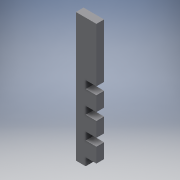
# Autodesk Inventor part: B
Saved by Autodesk Inventor 2019 (Build 230136000, 136)
## iProperties
Created: 2020-03-27
Part Number: B
Material: Generic
Document SubType Name: Modeling
Designer: Pulag
Density: 1 g/cm^3
Appearance: Default
Author: Pulag
Autodesk Inventor part; units mm, degrees
ref_plane "YZ Plane" through (0, 0, 0) normal (1, 0, 0) x (0, 1, 0)
ref_plane "XZ Plane" through (0, 0, 0) normal (0, 1, 0) x (-1, 0, 0)
ref_plane "XY Plane" through (0, 0, 0) normal (0, 0, 1) x (1, 0, 0)
sketch "Sketch1" plane through (0, 0, 0) normal (0, 0, 1) x (1, 0, 0)
  circle A0 centre (-2.5, 4.3301) radius 1.5 projected
  circle A1 centre (-2.5, -4.3301) radius 1.5 projected
  line L0 (-3.5898, 5.3609) -> (2.6004, 5.3609) construction
  line L1 (-2.5, -2.8301) -> (-6.6848, -2.8301)
  line L2 (-6.6848, -2.8301) -> (-6.6848, -5.8301)
  line L3 (-2.5, 5.8301) -> (-6.6848, 5.8301)
  line L4 (-2.5, 2.8301) -> (-6.6848, 2.8301)
  line L5 (-6.6848, 2.8301) -> (-6.6848, 5.8301)
  line L6 (-10.5, 44.1699) -> (-2.5, 44.1699)
  line L7 (-6.6848, -5.8301) -> (-10.5, -5.8301)
  line L8 (-10.5, -5.8301) -> (-10.5, 44.1699)
  line L9 (-6.6848, 0.0001) -> (-6.6849, 0)
  line L10 (-2.5, 2.8301) -> (-2.5, -2.8301)
  line L11 (-2.5, 14.4904) -> (-6.6848, 14.4904)
  line L12 (-2.5, 11.4904) -> (-6.6848, 11.4904)
  line L13 (-6.6848, 11.4904) -> (-6.6848, 14.4904)
  line L14 (-2.5, 11.4904) -> (-2.5, 5.8301)
  line L15 (-2.5, 23.1506) -> (-6.6848, 23.1506)
  line L16 (-2.5, 20.1506) -> (-6.6848, 20.1506)
  line L17 (-6.6848, 20.1506) -> (-6.6848, 23.1506)
  line L18 (-2.5, 20.1506) -> (-2.5, 14.4904)
  line L19 (-2.5, 11.4904) -> (-2.5, 5.8301)
  line L20 (-2.5, 44.1699) -> (-2.5, 23.1506)
  line L21 (-2.5, 20.1506) -> (-2.5, 14.4904)
  point P0 (0, 0)
  point P1 (-5.6848, 1.0001)
  constraints: 44 end point, 8 perpendicular, 6 horizontal, 5 parallel, 3 point on circle, 2 point on line, 1 vertical alignment, 1 other
extrude "Extrusion1" add sketch "Sketch1" along normal blind 3 contours L3 L5 L4 L10 L1 L2 L7 L8 L6 L20 L15 L17 L16 L18 L11 L13 L12 L14
body "Solid1"
